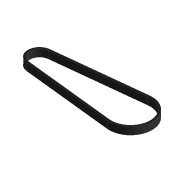
# Autodesk Inventor part: Conrod
Saved by Autodesk Inventor 2022.5 (Build 265521000, 521)
## iProperties
Created: 2018-04-07
Part Number: Conrod
Document SubType Name: Modeling
Designer: Administrator
Density: 1 g/cm^3
Mass: 2.37032 g
Surface Area: 28.3798 cm^2
Volume: 2.37032 cm^3
Material: Generic
Appearance: Rubber - Black
Author: Administrator
Autodesk Inventor part; units mm, degrees
ref_plane "YZ Plane" through (0, 0, 0) normal (1, 0, 0) x (0, 1, 0)
ref_plane "XZ Plane" through (0, 0, 0) normal (0, 1, 0) x (-1, 0, 0)
ref_plane "XY Plane" through (0, 0, 0) normal (0, 0, 1) x (1, 0, 0)
sketch "Sketch3" plane through (0, 0, 0) normal (0, 1, 0) x (-1, 0, 0)
  line L0 (0, 0) -> (8, 0) construction
  line L1 (8, 0) -> (8, -3)
  line L2 (8, -3) -> (9.5, -3)
  line L3 (9.5, -3) -> (9.5, 3)
  line L4 (9.5, 3) -> (8, 3)
  line L5 (8, 3) -> (8, 0)
  dimension "d9" = 1.5
  dimension "d10" = 6
  dimension "d11" = 8
  constraints: 12 end point, 5 perpendicular, 1 collinear, 1 horizontal, 1 point on line
  measures "d9" distance between parallel lines of L5 L3
  measures "d10" distance of L2.end L3.end
  measures "d11" distance from line of L0.start L5
sketch "Sketch1" plane through (0, 0, 0) normal (0, 0, 1) x (1, 0, 0)
  line L0 (0, 0) -> (74.5, 0) construction
  arc A0 (72.7819, -15.9075) -> (72.7819, 15.9075) centre (74.5, 0) ccw
  arc A1 (-0.8591, 7.9537) -> (-0.8591, -7.9537) centre (0, 0) ccw
  line L1 (-0.8591, 7.9537) -> (72.7819, 15.9075)
  line L2 (-0.8591, -7.9537) -> (72.7819, -15.9075)
  dimension "d0" = 74.5
  dimension "d2" = 16
  dimension "d8" = 32
  constraints: 6 end point, 4 point on circle, 2 centre point, 2 coincident, 2 symmetric about line, 2 tangent, 1 horizontal, 1 other
  measures "d0" distance of L0.start L0.end
  measures "d2" diameter of A1
  measures "d8" diameter of A0
sweep "Sweep1" add profiles "Sketch3" path "Sketch1"
body "Solid2"
